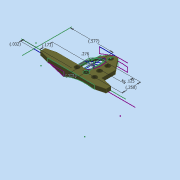
# Autodesk Inventor part: MPS Headpost
Saved by Autodesk Inventor 2012 SP2 (Build 160219200, 219)
## iProperties
Created: 2008-12-09
Part Number: MPS Headpost
Document SubType Name: Modeling
Designer: Ning-long Xu
Density: 4.51 g/cm^3
Material: Titanium
Description: Headpost
Mass: 0.602365 g
Surface Area: 3.42709 cm^2
Volume: 0.133562 cm^3
ALTERED ITEM PART NUMBER: N/A
ALTERED ITEM VENDOR: N/A
ALTERED ITEM DESCRIPTION: N/A
DESIGN DEPARTMENT: HHMI: JFRC - ID&F
LAB/DEPT: P-194005
REQUESTING SCIENTIST: Simon Peron
Revision Number: 0
Autodesk Inventor part; units mm, degrees
sketch "HeadplateSketch" plane through (0, 0, 0) normal (0, 0, 1) x (1, 0, 0)
  line L0 (22.2193, -2.4109) -> (25.4193, -1.6109)
  line L1 (25.4193, -1.6109) -> (25.4193, -0.0109)
  line L2 (6.3193, 0.7891) -> (3.1193, -0.0109)
  line L3 (3.1193, -1.6109) -> (3.1193, -0.0109)
  line L4 (6.3193, 0.7891) -> (22.2193, 0.7891)
  line L5 (22.2193, 0.7891) -> (25.4193, -0.0109)
  line L6 (17.1922, 9.6958) -> (17.1922, -2.4109)
  line L7 (17.1922, 9.6958) -> (18.128, 9.6958)
  line L8 (17.1922, 9.6958) -> (15.1602, 9.6958)
  line L9 (11.7996, 5.443) -> (11.7996, -2.4109)
  line L10 (21.4383, 5.5008) -> (21.4383, -2.4109)
  line L11 (21.4383, 5.5008) -> (18.128, 9.6958)
  arc A0 (15.1602, 9.6958) -> (11.7996, 5.443) centre (17.4689, 4.4173) ccw
  line L12 (3.1193, -1.6109) -> (6.3193, -2.4109)
  line L13 (6.3193, -2.4109) -> (22.2193, -2.4109)
  point P0 (11.7996, 0.7891)
  dimension "d95" = 3.2
  dimension "d102" = 1.6
  dimension "d104" = 3.2
  dimension "d106" = 0.8
  dimension "d109" = 1.6
  dimension "d110" = 3.2
  dimension "d112" = 22.3
  dimension "d113" = 15.9
  constraints: 29 end point, 5 point on line, 4 perpendicular, 3 parallel, 2 point on circle, 1 centre point, 1 horizontal
  measures "d95" horizontal distance of L2.start L2.end
  measures "d102" distance of L0.end L1.end
  measures "d104" horizontal distance of L0.start L0.end
  measures "d106" vertical distance of L1.end L4.end
  measures "d109" distance of L3.start L2.end
  measures "d110" horizontal distance of L4.end L1.end
  measures "d112" distance between parallel lines of L1 L3
  measures "d113" distance of L2.start L4.end
extrude "拉伸1" add sketch "HeadplateSketch" along normal blind 1.27
extrude "拉伸8" add sketch "HeadplateSketch" against normal blind 1.5 contours L13 L6 L4 L10 | L4 L6 L7 L11 L10 | L13 L9 L4 L6 | L4 L9 A0 L8 L6
sketch "草图2" plane through (15.1602, 9.6958, 1.27) normal (0, 1, 0) x (1, 0, 0)
  line L0 (-3.3633, 2.0352) -> (1.9994, 0)
  arc A0 (-3.3633, 2.77) -> (6.2787, 1.2693) centre (3.7754, 16.9113) ccw
  line L1 (1.9994, 0) -> (6.2787, 0)
  line L2 (-3.3633, 2.77) -> (6.2787, 2.77)
  line L3 (2.9678, 2.77) -> (0, 2.77) projected
  line L4 (6.2787, 1.2693) -> (6.2787, 2.77)
  line L5 (-3.3633, 0) -> (1.9994, 0)
  line L6 (0, 0) -> (2.9678, 0) projected
  line L7 (2.9678, 0) -> (2.9678, 2.77) projected
  line L8 (-3.3633, 0) -> (-3.3633, 2.0352)
  constraints: 12 end point, 2 point on circle, 2 point on line, 1 centre point, 1 parallel, 1 perpendicular
extrude "拉伸4" cut sketch "草图2" against normal up to next contours A0 L2 L7 | L7 L2 L4 A0
sketch "草图6" plane through (6.3193, -2.4109, 0) normal (0, -1, 0) x (1, 0, 0)
  line L0 (0, 0) -> (5.5435, 0)
  line L1 (0.6566, 0) -> (5.5435, -1.4987)
  line L2 (5.5435, 0) -> (5.5435, -1.4987)
  line L3 (0.6566, 0) -> (5.5435, 0)
  arc A0 (15.1197, 0.0007) -> (5.4803, -1.4987) centre (12.6164, -15.6413) ccw projected
  line L4 (15.1197, 0.0007) -> (15.1197, 0) projected
  line L5 (15.1197, 0) -> (15.9, 0) projected
  line L6 (15.9, 0) -> (15.9, 1.27) projected
  line L7 (15.9, 1.27) -> (0, 1.27) projected
  line L8 (0, 0) -> (0, 1.27) projected
  line L9 (0, 0) -> (5.4803, 0) projected
  line L10 (5.4803, 0) -> (5.4803, -1.4987) projected
  constraints: 8 end point, 1 perpendicular, 1 point on line
extrude "拉伸7" add sketch "草图6" against normal up to surface (3.2 mm away) contours L0 L10 L1 | L0 L2 A0 L1 L10 | A0 L2 L1
sketch "草图3" plane through (6.3193, 0.7891, 0) normal (0, 1, 0) x (1, 0, 0)
  line L0 (0, -1.27) -> (5.4803, -1.27) projected
  line L1 (5.4803, 0) -> (5.4803, -1.27) projected
  line L2 (5.4803, 0) -> (0, 0) projected
  line L3 (0, 0) -> (0, -1.27) projected
  line L4 (5.4803, -1.27) -> (16.1538, -1.27)
  line L5 (16.1538, -1.27) -> (17.1139, -1.27)
  line L6 (17.1139, -1.27) -> (17.1139, 0.0011)
  constraints: 6 end point, 2 perpendicular, 1 collinear
extrude "拉伸9" cut sketch "草图2" against normal up to surface (8.9067 mm away) contours L0 L5 L8
sketch "草图4" plane through (0, 0, 1.27) normal (0, 0, 1) x (1, 0, 0)
  circle A0 centre (17.2686, 8.053) radius 0.825
  circle A1 centre (18.9292, 5.4282) radius 0.825
  circle A2 centre (19.0006, 2.5892) radius 0.825
  circle A3 centre (17.1095, -0.097) radius 0.825
  line L0 (6.3193, 0.7891) -> (11.7996, 0.7891) projected
  line L1 (12.1356, 5.3815) -> (12.1356, 2.0023)
  line L2 (12.1356, 5.3815) -> (17.1561, 5.3815)
  line L3 (17.1561, 5.3815) -> (17.1561, 2.008)
  line L4 (17.1561, 2.008) -> (12.1356, 2.008)
  line L5 (11.7983, 4.0675) -> (12.1356, 4.0675)
  arc A4 (17.1561, 5.3815) -> (12.1356, 5.3815) centre (14.6459, 4.9584) ccw
  arc A5 (12.1356, 2.008) -> (17.1561, 2.008) centre (14.6459, 5.3033) ccw
  circle A6 centre (19.9896, -0.0785) radius 0.825
  circle A7 centre (14.1001, -0.1524) radius 0.825
  constraints: 10 end point, 8 centre point, 5 perpendicular, 4 point on circle, 2 point on line
extrude "拉伸10" cut sketch "草图4" against normal through all contours L2 L3 L4 L1 | A4 L2 | L4 A5
hole "打孔7" at (18.9292, 5.4282, 1.27) at (19.0006, 2.5892, 1.27) at (17.1095, -0.097, 1.27) at (17.2686, 8.053, 1.27) direction (0, 0, -1) diameter 1.65 end through all
hole "打孔8" at (14.1001, -0.1524, 1.27) at (19.9896, -0.0785, 1.27) direction (0, 0, -1) diameter 1.65 end through all
sketch "Sketch8" plane through (0, 0, 0) normal (0, 0, 1) x (1, 0, 0)
  arc A0 (17.1561, 5.3815) -> (12.1356, 5.3815) centre (14.6459, 4.9584) ccw projected
  arc A1 (12.1356, 2.008) -> (17.1561, 2.008) centre (14.6459, 5.3033) ccw projected
  line L0 (17.1596, 7.2353) -> (17.1596, 0.7891) projected
  line L1 (12.1356, 2.008) -> (12.1356, 5.3815) projected
  line L2 (14.6459, 7.5041) -> (14.6459, 1.1608)
  line L3 (17.1596, 4.3324) -> (12.1356, 4.3324)
  line L4 (-5.0839, 0) -> (30.5031, 0) projected
  line L5 (0, 12.1209) -> (0, -4.8328) projected
  point P0 (0, 0)
  dimension "d116" = 6.3433
  dimension "d117" = 3.1717
  dimension "d118" = 14.6459
  dimension "d119" = 4.3324
  constraints: 4 end point, 2 point on circle, 2 point on line, 1 parallel, 1 perpendicular
  measures "d116" distance of L2.start L2.end
  measures "d117" distance from line of L3 L2.start
  measures "d118" distance from line of A0.centre L5
  measures "d119" distance between parallel lines of L3 L4
sketch "Sketch9" plane through (11.7996, 0.7891, -0.7642) normal (-0.3548, 0, 0.9349) x (0.9349, 0, 0.3548)
  ellipse E0 centre (5.8496, 7.2639) end of major axis (6.7321, 7.2639) minor radius 0.825 (5.7331, 8.0816) -> (5.7331, 6.4461) ccw projected
  line L0 (5.7331, 8.9067) -> (5.7331, 8.0816) projected
  line L1 (3.5945, 8.9067) -> (5.7331, 8.9067) projected
  ellipse E1 centre (6.0638, 3.6282) end of major axis (-0.0984, 3.6282) minor radius 5.7613 (3.5945, 8.9067) -> (0, 4.6539) ccw projected
  line L2 (0, 0) -> (0, 4.6539) projected
  line L3 (0, 0) -> (5.7331, 0) projected
  line L4 (5.7331, 6.4461) -> (5.7331, 0) projected
  line L5 (5.7293, 4.5923) -> (5.7293, 1.2188) projected
  ellipse E2 centre (3.0444, 4.5141) end of major axis (-1.3864, 4.5141) minor radius 4.1425 (0.3594, 1.2188) -> (5.7293, 1.2188) ccw projected
  line L6 (0.3594, 1.2188) -> (0.3594, 4.5923) projected
  ellipse E3 centre (3.0444, 4.1693) end of major axis (5.7672, 4.1693) minor radius 2.5457 (5.7293, 4.5923) -> (0.3594, 4.5923) ccw projected
  line L7 (5.3145, 1.2188) -> (5.3145, 4.5923) projected
  arc A0 (0.112, 1.2188) -> (5.3145, 1.2188) centre (5.3145, 1.2188) ccw projected
  arc A1 (5.3145, 4.5923) -> (0.112, 4.5923) centre (0.112, 4.5923) ccw projected
  line L8 (5.3145, 4.5923) -> (0.3594, 4.5923)
  line L9 (2.8369, 6.7075) -> (4.6638, 6.7075)
  line L10 (2.8369, 0.3762) -> (5.3145, 0.3762)
  line L11 (2.8369, 6.7075) -> (2.8369, 0.3762)
  line L12 (2.8369, 3.5419) -> (5.3145, 3.5419)
  line L13 (2.9322, 6.7149) -> (2.9322, 0.3716) projected
  point P0 (-10.7607, -0.7891)
  dimension "d121" = 0.0953
  constraints: 10 end point, 3 perpendicular, 2 horizontal, 2 horizontal alignment, 1 midpoint, 1 point on line, 6 other
  measures "d121" distance between parallel lines of L13 L11
ref_plane "Work Plane3" through (11.7996, 0.7891, -0.7642) normal (-0.3548, 0, 0.9349) x (0.9349, 0, 0.3548)
ref_plane "Work Plane1" through (14.558, 0, 0) normal (1, 0, 0) x (0, 1, 0)
ref_plane "Work Plane2" through (0, 4.332, 0) normal (0, 1, 0) x (-1, 0, 0)
ref_plane "Work Plane4" through (0, 0, 0.283) normal (0, 0, 1) x (1, 0, 0)
sketch "Sketch10" plane through (0, 0, 0) normal (0, 0, 1) x (1, 0, 0)
  line L0 (3.1193, -1.6109) -> (3.1193, -0.0109) projected
  line L1 (3.1193, -0.8109) -> (0, -0.8109)
  line L2 (25.404, -0.8109) -> (34.4809, -0.8109)
  point P0 (0, 0)
  dimension "d126" = 0.8109
  constraints: 4 end point, 1 collinear, 1 midpoint, 1 perpendicular
  measures "d126" distance from line of point (0, 0) L1
ref_plane "Work Plane5" through (0, -0.811, 0) normal (0, 1, 0) x (-1, 0, 0)
sketch "Sketch11" plane through (11.7996, 0.7891, -0.7642) normal (-0.3548, 0, 0.9349) x (0.9349, 0, 0.3548)
  ellipse E0 centre (5.8496, 7.2639) end of major axis (6.7321, 7.2639) minor radius 0.825 (5.7331, 8.0816) -> (5.7331, 6.4461) ccw projected
  line L0 (5.7331, 8.9067) -> (5.7331, 8.0816) projected
  line L1 (3.5945, 8.9067) -> (5.7331, 8.9067) projected
  ellipse E1 centre (6.0638, 3.6282) end of major axis (-0.0984, 3.6282) minor radius 5.7613 (3.5945, 8.9067) -> (0, 4.6539) ccw projected
  line L2 (0, 0) -> (0, 4.6539) projected
  line L3 (0, 0) -> (5.7331, 0) projected
  line L4 (5.7331, 6.4461) -> (5.7331, 0) projected
  line L5 (5.7293, 4.5923) -> (5.7293, 1.2188) projected
  ellipse E2 centre (3.0444, 4.5141) end of major axis (-1.3864, 4.5141) minor radius 4.1425 (0.3594, 1.2188) -> (5.7293, 1.2188) ccw projected
  line L6 (0.3594, 1.2188) -> (0.3594, 4.5923) projected
  ellipse E3 centre (3.0444, 4.1693) end of major axis (5.7672, 4.1693) minor radius 2.5457 (5.7293, 4.5923) -> (0.3594, 4.5923) ccw projected
  circle A0 centre (3.0444, 3.5307) radius 3.5
  point P0 (-10.7607, -0.7891)
  dimension "d128" = 7
  constraints: 1 centre point, 4 other
  measures "d128" diameter of A0
ref_plane "Work Plane6" through (12.0474, 0.7891, -1.4172) normal (-0.3548, 0, 0.9349) x (0.9349, 0, 0.3548)
sketch "Sketch12" plane through (0, 0, 1.27) normal (0, 0, 1) x (1, 0, 0)
  circle A0 centre (17.1095, -0.097) radius 0.825 projected
  line L0 (14.541, 7.5041) -> (14.541, 1.1608) projected
  point P0 (0, 0)
  dimension "d130" = 2.5684
  measures "d130" distance from line of A0.centre L0
equation "\"d117\" = 0.5 * d116"
body "Solid1"
